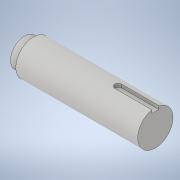
# Autodesk Inventor part: DTR-3
Saved by Autodesk Inventor 2021 (Build 250183000, 183)
## iProperties
Created: 2020-09-20
Part Number: DTR-3
Material: Generic
Document SubType Name: Modeling
Designer: Lucas Foulk
Density: 1 g/cm^3
Appearance: Default
Material_size: Steel
Quantity: 1
Author: Lucas Foulk
Autodesk Inventor part; units mm, degrees
ref_plane "YZ Plane" through (0, 0, 0) normal (1, 0, 0) x (0, 1, 0)
ref_plane "XZ Plane" through (0, 0, 0) normal (0, 1, 0) x (-1, 0, 0)
ref_plane "XY Plane" through (0, 0, 0) normal (0, 0, 1) x (1, 0, 0)
sketch "Sketch1" plane through (0, 0, 0) normal (1, 0, 0) x (0, 1, 0)
  circle A0 centre (0, 0) radius 15.875
  dimension "d0" = 31.75
  constraints: 1 centre point, 1 coincident
  measures "d0" diameter of A0
extrude "Extrusion1" add sketch "Sketch1" along normal blind 117.7036
ref_plane "Work Plane1" through (65.5447, 0, 0) normal (1, 0, 0) x (0, 0, -1)
sketch "Sketch9" plane through (117.7036, 0, 0) normal (1, 0, 0) x (0, 0, -1)
  line L0 (-3.175, 15.875) -> (-3.175, 12.7)
  line L1 (-3.175, 12.7) -> (3.175, 12.7)
  line L2 (3.175, 12.7) -> (3.175, 15.875)
  line L3 (0, 0) -> (0, 19.977)
  circle A0 centre (0, 0) radius 15.875 projected
  line L4 (0, 15.875) -> (-16.159, 15.875)
  point P0 (0, 12.7)
  point P1 (3.175, 15.5543)
  point P2 (-3.175, 15.5543)
  dimension "d26" = 6.35
  dimension "d27" = 3.175
  constraints: 10 end point, 2 horizontal, 2 perpendicular, 2 point on line, 2 vertical, 1 midpoint, 1 parallel, 2 other
  measures "d26" distance of L0.end L1.end
  measures "d27" distance between parallel lines of L1 L4
extrude "Extrusion9" cut sketch "Sketch9" against normal blind 33.3502 contours A0 L3 L1 L0 | A0 L2 L1 L3
sketch "Sketch10" plane through (0, 0, 0) normal (-1, 0, 0) x (0, 0, 1)
  circle A0 centre (0, 0) radius 15.875
  circle A1 centre (0, 0) radius 12.7
  dimension "d30" = 25.4
  constraints: 2 centre point, 2 coincident
  measures "d30" diameter of A1
extrude "Extrusion10" cut sketch "Sketch10" against normal blind 7.9375
sketch "Sketch11" plane through (117.7036, 12.7, 3.175) normal (0, 1, 0) x (1, 0, 0)
  line L0 (0, 0) -> (-33.3502, 0) projected
  line L1 (-33.3502, 6.35) -> (0, 6.35) projected
  line L2 (-33.3502, 6.35) -> (-33.3502, 0) projected
  arc A0 (-36.4412, 5.0705) -> (-33.3502, 0) centre (-39.0546, 0) ccw
  circle A1 centre (-33.3502, 3.175) radius 3.175
  point P0 (-117.7036, 3.175)
  constraints: 2 point on circle, 1 centre point, 1 midpoint, 1 tangent, 1 vertical alignment, 2 other
extrude "Extrusion11" cut sketch "Sketch11" along normal blind 25.4
body "Solid1"
